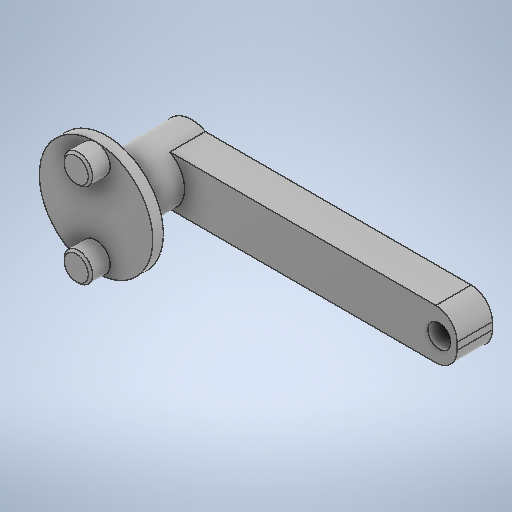
# Autodesk Inventor part: link_arm_1
Saved by Autodesk Inventor 2025 (Build 290162000, 162)
## iProperties
Created: 2025-09-10
Part Number: link_arm_1
Material: 一般
Document SubType Name: Modeling
Designer: sooo1
Density: 1 g/cm^3
Appearance: 滑らか - 標準の灰色
Author: sooo1
Autodesk Inventor part; units mm, degrees
ref_plane "YZ Plane" through (0, 0, 0) normal (1, 0, 0) x (0, 1, 0)
ref_plane "XZ Plane" through (0, 0, 0) normal (0, 1, 0) x (-1, 0, 0)
ref_plane "XY Plane" through (0, 0, 0) normal (0, 0, 1) x (1, 0, 0)
sketch "スケッチ1" plane through (0, 0, 0) normal (0, 0, 1) x (1, 0, 0)
  line L0 (-22.5, 3.5) -> (22.5, 3.5)
  line L1 (22.5, 3.5) -> (22.5, -3.5)
  line L2 (22.5, -3.5) -> (-22.5, -3.5)
  line L3 (-22.5, -3.5) -> (-22.5, 3.5)
  line L4 (-22.5, 3.5) -> (22.5, -3.5) construction
  line L5 (22.5, 3.5) -> (-22.5, -3.5) construction
  line L6 (0, -11.2) -> (0, 11.2) construction
  line L7 (-38.51, 0) -> (35.06, 0) construction
  circle A0 centre (-20, 0) radius 4.55
  line L8 (22.5, -3.5) -> (22.5, 3.5)
  circle A1 centre (20, 0) radius 4.55
  circle A2 centre (20, 0) radius 1.6
  circle A3 centre (-20, 0) radius 1
  circle A4 centre (-20, 0) radius 4
  line L9 (-20, 4) -> (-20, -4) construction
  circle A5 centre (-20, 6) radius 2
  circle A6 centre (-20, -6) radius 2
  circle A7 centre (-20, 0) radius 4
  circle A8 centre (-20, 0) radius 8
  point P0 (0, 0)
  point P1 (-17.0927, 3.5)
  point P2 (-22.9073, 3.5)
  point P3 (-22.9073, -3.5)
  point P4 (-17.0927, -3.5)
  point P5 (17.0927, 3.5)
  point P6 (17.0927, -3.5)
  point P7 (22.9073, -3.5)
  point P8 (22.9073, 3.5)
  dimension "d1" = 7
  dimension "d2" = 20
  dimension "d3" = 45
  dimension "d4" = 9.1
  dimension "d13" = 3.2
  dimension "d14" = 2
  dimension "d15" = 8
  dimension "d16" = 4
  dimension "d17" = 4
  dimension "d18" = 12
  constraints: 16 end point, 9 centre point, 5 coincident, 4 midpoint, 4 point on line, 3 tangent, 2 parallel, 2 point on circle, 1 horizontal, 1 perpendicular, 1 symmetric about line, 1 vertical, 1 other
  measures "d1" distance of L2.end L0.start
  measures "d2" distance from line of L6 A0.centre
  measures "d3" distance of L0.start L0.end
  measures "d4" diameter of A0
  measures "d13" diameter of A2
  measures "d14" diameter of A3
  measures "d15" diameter of A4
  measures "d16" diameter of A5
  measures "d17" diameter of A6
  measures "d18" distance of A6.centre A5.centre
extrude "押し出し1" add sketch "スケッチ1" along normal mid plane 5 contours L0 A4 L3 | L0 A4 L2 L3 | L0 A0 L2 A4 | A4 L2 L3 | L0 A8 L2 A0 | L0 A1 L2 A8 | L0 L1 L2 A1 picked at (19.7999, -2.8628)
fillet "フィレット1" radius 3 4 edges at (-22.5, 3.5, 0) (-22.5, -3.5, 0) (22.5, -3.5, 0) (22.5, 3.5, 0)
extrude "押し出し3" add sketch "スケッチ1" along normal blind 11 from surface at -2.5 contours A4 L0 | L0 A4 L2 L3 | L3 A4 | L2 A4
extrude "押し出し5" add sketch "スケッチ1" along normal blind 1 from surface at 8.5 contours A4 L0 | L0 A4 L2 L3 | L3 A4 | L2 A4 | A3
extrude "押し出し6" add sketch "スケッチ1" along normal blind 1.5 from surface at 9.5 contours L3 A4 L2 A6 A0 A5 L0 | L0 A4 L3 | A4 L0 | L0 A4 L2 L3 | L3 A4 | A4 A5 A0 L0 | L0 A0 L2 A4 | A5 A0 | A4 L2 L3 | A0 A5 A8 L0 | L0 A8 L2 A0 | A5 A0 | A0 A6 A8 A5 | L2 A4 | L2 A0 A6 A4 | A6 A0 | A0 A6 | L2 A8 A6 A0 | A3
extrude "押し出し7" add sketch "スケッチ1" along normal blind 2.8 from surface at 11 contours A5 A0 | A5 A0 | A6 A0 | A0 A6
chamfer "面取り1" distance 0.3 angle 45 2 edges at (-22, 6, 13.8) (-22, -6, 13.8)
